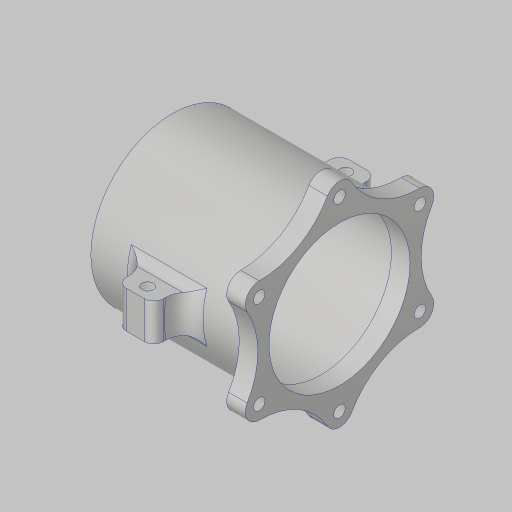
# Autodesk Inventor part: AR-010
Saved by Autodesk Inventor 2023.5 (Build 275446000, 446)
## iProperties
Created: 2025-01-24
Part Number: AR-010
Material: Aluminum 6061
Document SubType Name: Modeling
Designer: slick
Density: 2.7 g/cm^3
Appearance: Aluminum - Flat
Author: slick
Autodesk Inventor part; units mm, degrees
ref_plane "YZ Plane" through (0, 0, 0) normal (1, 0, 0) x (0, 1, 0)
ref_plane "XZ Plane" through (0, 0, 0) normal (0, 1, 0) x (-1, 0, 0)
sketch "Sketch1" plane through (0, 0, 0) normal (1, 0, 0) x (0, 1, 0)
  circle A0 centre (0, 0) radius 25.4
  circle A1 centre (0, 0) radius 27.94
  dimension "d0" = 50.8
  dimension "d1" = 2.54
  constraints: 2 centre point, 1 coincident
  measures "d0" diameter of A0
  measures "d1" radial gap between concentric circles of A0 A1
extrude "Extrusion1" add sketch "Sketch1" along normal mid plane 50.8
sketch "Sketch2" plane through (25.4, 0, 0) normal (1, 0, 0) x (0, 0, -1)
  line L0 (38.1, -38.1) -> (-38.1, -38.1) construction
  line L1 (-38.1, -38.1) -> (-38.1, 38.1) construction
  line L2 (-38.1, 38.1) -> (38.1, 38.1) construction
  line L3 (38.1, 38.1) -> (38.1, -38.1) construction
  line L4 (38.1, -38.1) -> (-38.1, 38.1) construction
  line L5 (-38.1, -38.1) -> (38.1, 38.1) construction
  circle A0 centre (0, 0) radius 38.1
  circle A1 centre (0, 0) radius 24.13
  dimension "d4" = 76.2
  dimension "d5" = 76.2
  dimension "d20" = 76.2
  dimension "d42" = 48.26
  constraints: 12 end point, 2 centre point, 2 coincident, 2 midpoint, 2 parallel, 1 horizontal, 1 perpendicular
  measures "d4" distance of L1.end L2.end
  measures "d5" distance of L0.end L1.end
  measures "d20" diameter of A0
  measures "d42" diameter of A1
extrude "Extrusion2" add sketch "Sketch2" along normal blind 6.35
sketch "Sketch3" plane through (31.75, 0, 0) normal (1, 0, 0) x (0, 0, -1)
  point P0 (0, 0)
  point P1 (0, 31.75)
  point P2 (-27.4963, 15.875)
  point P3 (-27.4963, -15.875)
  point P4 (0, -31.75)
  point P5 (27.4963, -15.875)
  point P6 (27.4963, 15.875)
  dimension "d8" = 31.75
  dimension "d11" = 360
  constraints: 1 vertical alignment, 7 other
  measures "d8" distance of point (0, 0) point (0, 31.75)
hole "Hole1" at (31.75, 31.75, 0) at (31.75, 15.875, 27.4963) at (31.75, -15.875, 27.4963) at (31.75, -31.75, 0) at (31.75, -15.875, -27.4963) at (31.75, 15.875, -27.4963) direction (-1, 0, 0) diameter 3.9624 end through all thread size "10-32 UNF" class "2B" standard "ANSI Unified Screw Threads"
ref_plane "Work Plane2" through (0, 0, 38.1) normal (0, 0, 1) x (1, 0, 0)
sketch "Sketch6" plane through (0, 0, 38.1) normal (0, 0, 1) x (1, 0, 0)
  line L0 (6.35, -6.35) -> (-6.35, -6.35)
  line L1 (-6.35, -6.35) -> (-6.35, 6.35)
  line L2 (-6.35, 6.35) -> (6.35, 6.35)
  line L3 (6.35, 6.35) -> (6.35, -6.35)
  line L4 (6.35, -6.35) -> (-6.35, 6.35) construction
  line L5 (-6.35, -6.35) -> (6.35, 6.35) construction
  point P0 (0, 0)
  dimension "d27" = 12.7
  dimension "d28" = 12.7
  constraints: 12 end point, 2 midpoint, 2 parallel, 1 horizontal, 1 perpendicular
  measures "d27" distance of L1.end L2.end
  measures "d28" distance of L0.end L1.end
extrude "Extrusion4" add sketch "Sketch6" against normal blind 12.7
mirror "Mirror1" about plane through (0, 0, 0) normal (0, 0, 1) of "Extrusion4"
fillet "Fillet1" radius 6.604 4 edges at (-6.35, 0, -27.94) (6.35, 0, -27.94) (-6.35, 0, 27.94) (6.35, 0, 27.94)
fillet "Fillet2" radius 3.302 16 edges at (-9.652, 6.35, 27.2088) (0, 6.35, 27.2088) (9.652, 6.35, 27.2088) (-9.652, 6.35, -27.2088) (0, 6.35, -27.2088) (9.652, 6.35, -27.2088) (9.652, -6.35, -27.2088) (0, -6.35, -27.2088) (-9.652, -6.35, -27.2088) (-9.652, -6.35, 27.2088) (0, -6.35, 27.2088) (9.652, -6.35, 27.2088) (-6.35, 0, -38.1) (6.35, 0, -38.1) (-6.35, 0, 38.1) (6.35, 0, 38.1)
sketch "Sketch7" plane through (-3.048, 6.35, -38.1) normal (0, 1, 0) x (1, 0, 0)
  line L0 (-22.352, -65.3088) -> (-22.352, -62.6934) projected
  line L1 (-22.352, -10.8912) -> (-9.906, -10.8912) projected
  line L2 (-4.7765, -8.3863) -> (10.8725, -8.3863) projected
  line L3 (9.398, -3.302) -> (9.398, -4.1447) projected
  arc A0 (9.398, -3.302) -> (6.096, 0) centre (6.096, -3.302) ccw projected
  line L4 (0, 0) -> (6.096, 0) projected
  arc A1 (0, 0) -> (-3.302, -3.302) centre (0, -3.302) ccw projected
  line L5 (-3.302, -4.1447) -> (-3.302, -3.302) projected
  line L6 (-22.352, -62.6934) -> (28.448, -62.6934) projected
  line L7 (28.448, -13.5066) -> (-22.352, -13.5066) projected
  line L8 (-22.352, -13.5066) -> (-22.352, -10.8912) projected
  line L9 (-9.906, -65.3088) -> (-22.352, -65.3088) projected
  line L10 (10.8725, -67.8137) -> (-4.7765, -67.8137) projected
  line L11 (9.398, -72.0553) -> (9.398, -72.898) projected
  arc A2 (6.096, -76.2) -> (9.398, -72.898) centre (6.096, -72.898) ccw projected
  line L12 (6.096, -76.2) -> (0, -76.2) projected
  arc A3 (-3.302, -72.898) -> (0, -76.2) centre (0, -72.898) ccw projected
  line L13 (-3.302, -72.898) -> (-3.302, -72.0553) projected
  line L14 (16.002, -10.8912) -> (28.448, -10.8912) projected
  line L15 (28.448, -75.6671) -> (28.448, -65.3088) projected
  line L16 (34.798, -75.6671) -> (28.448, -75.6671) projected
  line L17 (28.448, -0.5329) -> (34.798, -0.5329) projected
  line L18 (28.448, -10.8912) -> (28.448, -0.5329) projected
  line L19 (28.448, -65.3088) -> (16.002, -65.3088) projected
  line L20 (6.096, -3.302) -> (0, -3.302) construction
  line L21 (6.096, -72.898) -> (0, -72.898) construction
  line L22 (28.448, -62.6934) -> (28.448, -61.3795) projected
  line L23 (28.448, -61.3795) -> (34.798, -61.3795) projected
  line L24 (34.798, -61.3795) -> (34.798, -75.6671) projected
  line L25 (28.448, -14.8205) -> (28.448, -13.5066) projected
  line L26 (34.798, -14.8205) -> (28.448, -14.8205) projected
  line L27 (34.798, -0.5329) -> (34.798, -14.8205) projected
  line L28 (3.048, -76.2) -> (3.048, -67.8137) construction
  line L29 (10.8725, -67.8137) -> (-4.7765, -67.8137) projected
  line L30 (3.048, 0) -> (3.048, -8.3863) construction
  point P0 (3.048, -38.1)
  point P1 (3.048, -72.0068)
  point P2 (3.048, -4.1932)
  point P3 (3.048, -3.302)
  point P4 (3.048, -72.0068)
  point P5 (3.048, -4.1932)
  constraints: 8 end point, 7 midpoint, 2 coincident, 2 horizontal, 2 vertical alignment, 8 other
hole "Hole2" at (0, 6.35, 33.9068) at (0, 6.35, -33.9068) direction (0, -1, 0) diameter 3.9624 end through all thread size "10-32 UNF" class "2B" standard "ANSI Unified Screw Threads"
sketch "Sketch8" plane through (31.75, 0, 0) normal (1, 0, 0) x (0, 0, -1)
  circle A0 centre (27.4963, -15.875) radius 1.9812 projected
  circle A1 centre (-27.4963, -15.875) radius 1.9812 projected
  circle A2 centre (0, 31.75) radius 1.9812 projected
  circle A3 centre (-27.4963, 15.875) radius 1.9812 projected
  circle A4 centre (0, -31.75) radius 1.9812 projected
  circle A5 centre (27.4963, 15.875) radius 1.9812 projected
  circle A6 centre (0, 0) radius 24.13 projected
  circle A7 centre (0, 0) radius 38.1 projected
  circle A8 centre (0, 31.75) radius 1.9812 construction
  circle A9 centre (0, 31.75) radius 4.7625 construction
  circle A10 centre (27.4963, 15.875) radius 4.7625 construction
  circle A11 centre (27.4963, -15.875) radius 4.7625 construction
  circle A12 centre (0, -31.75) radius 4.7625 construction
  circle A13 centre (-27.4963, -15.875) radius 1.9812 construction
  circle A14 centre (-27.4963, -15.875) radius 4.7625 construction
  circle A15 centre (-27.4963, 15.875) radius 1.9812 construction
  circle A16 centre (-27.4963, 15.875) radius 4.7625 construction
  arc A17 (-27.4599, 20.6374) -> (-4.1425, 34.0996) centre (-27.2567, 47.21) ccw
  arc A18 (4.1425, 34.0996) -> (27.4599, 20.6374) centre (27.2567, 47.21) ccw
  circle A19 centre (27.4963, -15.875) radius 1.9812 construction
  circle A20 centre (-27.4963, -15.875) radius 1.9812 construction
  circle A21 centre (0, 31.75) radius 1.9812 construction
  circle A22 centre (-27.4963, 15.875) radius 1.9812 construction
  circle A23 centre (0, -31.75) radius 1.9812 construction
  circle A24 centre (27.4963, 15.875) radius 1.9812 construction
  circle A25 centre (0, 0) radius 24.13 construction
  circle A26 centre (0, 0) radius 38.1 construction
  circle A27 centre (0, 0) radius 27.94 construction
  arc A28 (31.6024, 13.4623) -> (31.6024, -13.4623) centre (54.5134, 0) ccw
  arc A29 (27.4599, -20.6374) -> (4.1425, -34.0996) centre (27.2567, -47.21) ccw
  arc A30 (-4.1425, -34.0996) -> (-27.4599, -20.6374) centre (-27.2567, -47.21) ccw
  arc A31 (-31.6024, -13.4623) -> (-31.6024, 13.4623) centre (-54.5134, 0) ccw
  arc A32 (4.1425, 34.0996) -> (-4.1425, 34.0996) centre (0, 31.75) ccw
  circle A33 centre (27.4963, 15.875) radius 1.9812 projected
  arc A34 (31.6024, 13.4623) -> (27.4599, 20.6374) centre (27.4963, 15.875) ccw
  arc A35 (27.4599, -20.6374) -> (31.6024, -13.4623) centre (27.4963, -15.875) ccw
  arc A36 (-4.1425, -34.0996) -> (4.1425, -34.0996) centre (0, -31.75) ccw
  arc A37 (-31.6024, -13.4623) -> (-27.4599, -20.6374) centre (-27.4963, -15.875) ccw
  arc A38 (-27.4599, 20.6374) -> (-31.6024, 13.4623) centre (-27.4963, 15.875) ccw
  point P0 (-31.6024, 13.4623)
  point P1 (31.6024, -13.4623)
  dimension "d43" = 9.525
  constraints: 37 point on circle, 18 centre point, 18 tangent, 12 coincident, 6 equal radius
  measures "d43" diameter of A9
extrude "Extrusion5" cut sketch "Sketch8" against normal up to surface (6.35 mm away) contours A7
body "Solid1"
